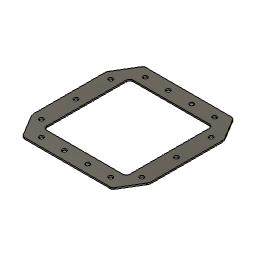
Motor_Mount_Backing_Plate v1 (Autodesk Fusion 360 design; units mm, degrees)
Autodesk Fusion 360 part; units mm, degrees
sketch "Sketch1" plane through (0, 0, 0) normal (0, 0, 1) x (1, 0, 0)
  line L0 (66.0529, 87.5864) -> (83.5676, 58.5358)
  line L1 (85.0032, 53.4602) -> (85.0032, -48.3705)
  arc A0 (85.0032, 53.4602) -> (83.5676, 58.5358) centre (75.0036, 53.3726) ccw
  line L2 (-0.008, -87.5) -> (0.0209, -87.5)
  line L3 (0.0209, 90.0048) -> (0.0209, -60.0001)
  line L4 (85.0032, 0) -> (60.0032, 0) construction
  line L5 (60.0032, 0) -> (60.0032, 60.0048)
  line L6 (60.0032, 0) -> (60.0032, -55.0001)
  line L7 (0, 2.5) -> (0, 20)
  line L8 (-66.0529, 87.5864) -> (-83.5676, 58.5358)
  arc A1 (-83.5676, 58.5358) -> (-85.0032, 53.4602) centre (-75.0036, 53.3726) ccw
  line L9 (-85.0032, 53.4602) -> (-85.0019, -48.3728)
  line L10 (-60.0032, 0) -> (-59.9614, 60.0083)
  line L11 (-60.0032, 0) -> (-60.0023, -55.0002)
  line L12 (0.008, -87.5) -> (-0.008, -87.5)
  line L13 (-54.9614, 65.0048) -> (55.0032, 65.0048)
  line L14 (-55.0023, -60.0001) -> (55.0032, -60.0001)
  arc A2 (-54.9614, 65.0048) -> (-59.9614, 60.0083) centre (-54.9614, 60.0048) ccw
  arc A3 (60.0032, 60.0048) -> (55.0032, 65.0048) centre (55.0032, 60.0048) ccw
  arc A4 (55.0032, -60.0001) -> (60.0032, -55.0001) centre (55.0032, -55.0001) ccw
  arc A5 (-60.0023, -55.0002) -> (-55.0023, -60.0001) centre (-55.0023, -55.0001) ccw
  line L15 (26.5988, -60.0001) -> (26.5988, -85.0001) construction
  line L16 (61.771, -85.0002) -> (-61.771, -85.0002)
  line L17 (0.0209, 65.0048) -> (0.0209, 90.0048)
  line L18 (61.7709, 90.0048) -> (-61.7709, 90.0048)
  arc A6 (-61.7709, 90.0048) -> (-66.0529, 87.5864) centre (-61.7709, 85.0048) ccw
  arc A7 (66.0529, 87.5864) -> (61.7709, 90.0048) centre (61.7709, 85.0048) ccw
  circle A8 centre (0.0209, 77.5048) radius 3 construction
  circle A9 centre (-49.9791, 77.5048) radius 3
  circle A10 centre (50.0209, 77.5048) radius 3
  circle A11 centre (72.5032, 0) radius 3
  circle A12 centre (72.5032, -50) radius 3
  circle A13 centre (72.5032, 50) radius 3
  circle A14 centre (-72.4614, 50) radius 3
  circle A15 centre (-72.4614, 0) radius 3
  circle A16 centre (-72.4614, -50) radius 3
  line L19 (0.0209, 65.0048) -> (0.0209, 2.5023)
  line L20 (0.0209, 2.5023) -> (60.0032, 2.5023)
  circle A17 centre (0.0209, -72.5002) radius 3 construction
  circle A18 centre (50.0209, -72.5002) radius 3
  circle A19 centre (-49.9791, -72.5002) radius 3
  line L21 (-83.5657, -53.5361) -> (-66.0529, -82.5819)
  line L22 (83.567, -53.5339) -> (66.0529, -82.5819)
  arc A20 (-83.5657, -53.5361) -> (-85.0019, -48.3728) centre (-75.0019, -48.3727) cw
  arc A21 (85.0032, -48.3705) -> (83.567, -53.5339) centre (75.0032, -48.3705) cw
  arc A22 (61.771, -85.0002) -> (66.0529, -82.5819) centre (61.771, -80.0002) ccw
  arc A23 (-66.0529, -82.5819) -> (-61.771, -85.0002) centre (-61.771, -80.0002) ccw
  line L23 (0.0209, 77.5048) -> (17.0209, 77.5048) construction
  line L24 (17.0209, 77.5048) -> (15, 77.5048) construction
  circle A24 centre (17.0209, 77.5048) radius 3
  circle A25 centre (-16.9791, 77.5048) radius 3
  circle A26 centre (-16.9791, -72.5002) radius 3
  circle A27 centre (17.0209, -72.5002) radius 3
  point P0 (-27.4888, 87.5035)
  point P1 (0.0209, 0)
  point P2 (72.5419, -75.2372)
  point P3 (60.0032, 65)
  point P4 (60.0032, -60)
  point P5 (85.0014, -85)
  point P6 (-85.0032, -51.1519)
  dimension "d13" = 10
  dimension "d21" = 65
  dimension "d22" = 60
  dimension "d23" = 5
  dimension "d25" = 25
  dimension "d28" = 25
  dimension "d29" = 5
  dimension "d30" = 6
  dimension "d33" = 50
  dimension "d34" = 0
  dimension "d35" = 6
  dimension "d38" = 0
  dimension "d39" = 50
  dimension "d40" = 62.5025
  dimension "d43" = 25
  dimension "d44" = 10
  dimension "d45" = 5
  dimension "d48" = 17
  dimension "d49" = 6
  constraint tangent L0 A0
  constraint vertical L1
  constraint horizontal L2
  constraint vertical L3
  constraint coincident P1 L3
  constraint coincident L1 L4.start
  constraint perpendicular L1 L4
  constraint vertical L5
  constraint vertical L6
  constraint symmetric L0.end L7 L8.end
  constraint symmetric L1.start L7 A1.end
  constraint symmetric L2.start L7 L12.start
  constraint symmetric A0 L7 A1
  constraint symmetric L4.end L7 L10.start
  constraint horizontal L13
  constraint horizontal L14
  constraint tangent L10 A2
  constraint tangent L13 A2
  constraint coincident P3 L5
  constraint tangent L13 A3
  constraint tangent L5 A3
  constraint equal A2 A3
  constraint coincident P4 L6
  constraint tangent L14 A4
  constraint tangent L6 A4
  constraint equal A2 A4
  constraint tangent L11 A5
  constraint tangent L14 A5
  constraint equal A2 A5
  constraint vertical L15
  constraint coincident L14 L15.start
  constraint horizontal L16
  constraint vertical L17
  constraint midpoint L13 L17.start
  constraint coincident L3.start L17.end
  constraint coincident L14 L3.end
  constraint horizontal L18
  constraint tangent L8 A6
  constraint tangent L18 A6
  constraint tangent L0 A7
  constraint tangent L18 A7
  constraint equal A6 A7
  constraint midpoint L17 A8.centre
  constraint midpoint L4 A11.centre
  constraint symmetric L3 A11 A15
  constraint symmetric L3 A12 A16
  constraint symmetric L3 A13 A14
  constraint perpendicular L14 L19
  constraint coincident L5 L20.end
  constraint perpendicular L5 L20
  constraint symmetric A8 L20 A17
  constraint symmetric A9 L20 A19
  constraint symmetric A10 L20 A18
  constraint tangent L9 A20
  constraint tangent L21 A20
  constraint tangent L22 A21
  constraint tangent L1 A21
  constraint equal A20 A21
  constraint tangent L22 A22
  constraint tangent L16 A22
  constraint tangent L16 A23
  constraint tangent L21 A23
  constraint equal A22 A23
  constraint horizontal L23
  constraint coincident A8.centre L23.start
  constraint coincident L23 L24.end
  constraint perpendicular L3 L24
  constraint coincident L23.end L24.start
  constraint symmetric L3 A24 A25
  constraint symmetric L20 A24 A27
  constraint symmetric L20 A25 A26
  measures "d13" radius of A0
  measures "d21" distance of L4.end P3
  measures "d22" distance of L4.end P4
  measures "d23" radius of A2
  measures "d25" distance of L15.start L15.end
  measures "d28" distance of L17.start L3.start
  measures "d29" radius of A6
  measures "d30" diameter of A8
  measures "d35" diameter of A11
  measures "d40" distance of L17.start L19.end
  measures "d43" distance of L1 L6
  measures "d44" radius of A20
  measures "d45" radius of A22
  measures "d48" distance of A8.centre L23.end
  measures "d49" diameter of A24
extrude "Extrude1" add sketch "Sketch1" along normal blind 2
chamfer "Chamfer1" [suppressed]
equation "d40 = ( 125.005 / 2 ) * 1 mm"
